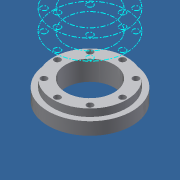
# Autodesk Inventor part: RotGear_spacer
Saved by Autodesk Inventor 2016 (Build 200138000, 138)
## iProperties
Created: 2016-03-29
Part Number: RotGear_spacer
Material: ABS-Kunststoff
Document SubType Name: Modeling
Designer: 4ndreas
Density: 1.06 g/cm^3
Appearance: Glatt - weiß
Mass: 6.80837 g
Surface Area: 41.1077 cm^2
Volume: 6.42299 cm^3
Author: 4ndreas
Autodesk Inventor part; units mm, degrees
ref_plane "YZ Plane" through (0, 0, 0) normal (1, 0, 0) x (0, 1, 0)
ref_plane "XZ Plane" through (0, 0, 0) normal (0, 1, 0) x (-1, 0, 0)
ref_plane "XY Plane" through (0, 0, 0) normal (0, 0, 1) x (1, 0, 0)
sketch "Skizze1" plane through (0, 0, 0) normal (0, 0, 1) x (1, 0, 0)
  circle A0 centre (-15.5, 0) radius 1.5 projected
  circle A1 centre (0, -15.5) radius 1.5 projected
  circle A2 centre (10.9602, 10.9602) radius 1.5 projected
  circle A3 centre (0, 15.5) radius 1.5 projected
  circle A4 centre (15.5, 0) radius 1.5 projected
  circle A5 centre (10.9602, -10.9602) radius 1.5 projected
  circle A6 centre (-10.9602, -10.9602) radius 1.5 projected
  circle A7 centre (-10.9602, 10.9602) radius 1.5 projected
  circle A8 centre (0, 0) radius 11.5 projected
  arc A9 (22.1589, -22.3882) -> (22.1589, 22.3882) centre (0, 0) ccw projected
  arc A10 (22.1589, 22.3882) -> (22.1589, -22.3882) centre (0, 0) ccw projected
  circle A11 centre (0, 0) radius 17.5
  point P0 (0, 0)
  dimension "d0" = 35
  constraints: 1 centre point, 1 coincident
  measures "d0" diameter of A11
extrude "Extrusion1" add sketch "Skizze1" along normal blind 9.5 contours A11
sketch "Skizze2" plane through (0, 0, 0) normal (0, 0, -1) x (-1, 0, 0)
  circle A0 centre (0, 0) radius 17.5 projected
  circle A1 centre (0, 0) radius 20
  point P0 (0, 0)
  dimension "d4" = 40
  constraints: 1 centre point, 1 coincident
  measures "d4" diameter of A1
extrude "Extrusion2" add sketch "Skizze2" against normal blind 6
